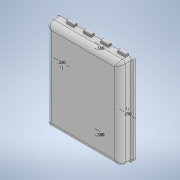
# Autodesk Inventor part: Top
Saved by Autodesk Inventor 2022 (Build 260153000, 153)
## iProperties
Created: 2022-03-05
Part Number: Top
Material: Generic
Document SubType Name: Modeling
Designer: Stump
Density: 1 g/cm^3
Appearance: Default
Author: Stump
Autodesk Inventor part; units mm, degrees
ref_plane "XZ Plane" through (0, 0, 0) normal (0, 1, 0) x (-1, 0, 0)
sketch "Sketch1" plane through (0, 0, 0) normal (0, 0, 1) x (1, 0, 0)
  line L0 (0, 0) -> (177.9524, 0)
  line L1 (177.9524, 0) -> (177.9524, 218.44)
  line L2 (177.9524, 218.44) -> (0, 218.44)
  line L3 (0, 218.44) -> (0, 0)
  line L4 (12.7, 205.74) -> (165.2524, 205.74)
  line L5 (165.2524, 205.74) -> (165.2524, 12.7)
  line L6 (165.2524, 12.7) -> (12.7, 12.7)
  line L7 (12.7, 12.7) -> (12.7, 205.74)
  dimension "d0" = 177.9524
  dimension "d1" = 218.44
  dimension "d2" = 12.7
  constraints: 16 end point, 4 parallel, 2 perpendicular, 1 horizontal, 3 other
  measures "d0" distance of L2.end L1.end
  measures "d1" distance of L1.end L0.end
  measures "d2" distance between parallel lines of L2 L4
extrude "Extrusion1" add sketch "Sketch1" along normal blind 28.194
sketch "Sketch2" plane through (0, 0, 28.194) normal (0, 0, 1) x (1, 0, 0)
  line L0 (177.9524, 0) -> (177.9524, 218.44) projected
  line L1 (177.9524, 218.44) -> (0, 218.44) projected
  line L2 (0, 218.44) -> (0, 0) projected
  line L3 (0, 0) -> (177.9524, 0) projected
  line L4 (12.7, 205.74) -> (165.2524, 205.74) projected
  line L5 (165.2524, 205.74) -> (165.2524, 12.7) projected
  line L6 (165.2524, 12.7) -> (12.7, 12.7) projected
  line L7 (12.7, 12.7) -> (12.7, 205.74) projected
  line L8 (0, 218.44) -> (0, 0) projected
  line L9 (0, 0) -> (177.9524, 0) projected
  line L10 (0, 218.44) -> (177.9524, 218.44)
  line L11 (177.9524, 218.44) -> (177.9524, 0)
  line L12 (177.9524, 0) -> (0, 0)
  line L13 (0, 0) -> (0, 218.44)
  constraints: 8 end point, 2 parallel, 1 horizontal, 1 perpendicular
extrude "Extrusion2" add sketch "Sketch2" against normal blind 3.175 contours L4 L5 L6 L7
fillet "Fillet1" radius 3.175 4 edges at (88.9762, 205.74, 25.019) (165.2524, 109.22, 25.019) (88.9762, 12.7, 25.019) (12.7, 109.22, 25.019)
fillet "Fillet3" radius 12.7 4 edges at (88.9762, 218.44, 28.194) (177.9524, 109.22, 28.194) (88.9762, 0, 28.194) (0, 109.22, 28.194)
fillet "Fillet4" radius 6.35 8 edges at (3.7197, 3.7197, 24.4743) (0, 0, 7.747) (174.2327, 3.7197, 24.4743) (177.9524, 0, 7.747) (3.7197, 214.7203, 24.4743) (0, 218.44, 7.747) (174.2327, 214.7203, 24.4743) (177.9524, 218.44, 7.747)
sketch "Sketch4" plane through (0, 0, 0) normal (0, 0, -1) x (-1, 0, 0)
  arc A0 (-177.9524, 6.35) -> (-171.6024, 0) centre (-171.6024, 6.35) ccw projected
  line L0 (0, 212.09) -> (0, 6.35) projected
  line L1 (0, 6.35) -> (0, 212.09)
  line L2 (-177.9524, 212.09) -> (-177.9524, 6.35)
  arc A1 (-171.6024, 218.44) -> (-177.9524, 212.09) centre (-171.6024, 212.09) ccw projected
  arc A2 (-171.6024, 218.44) -> (-177.9524, 212.09) centre (-171.6024, 212.09) ccw
  arc A3 (0, 212.09) -> (-6.35, 218.44) centre (-6.35, 212.09) ccw projected
  line L3 (-171.6024, 218.44) -> (-6.35, 218.44) projected
  arc A4 (0, 212.09) -> (-6.35, 218.44) centre (-6.35, 212.09) ccw
  line L4 (-177.9524, 6.35) -> (-177.9524, 212.09) projected
  line L5 (-6.35, 0) -> (-171.6024, 0) projected
  arc A5 (-177.9524, 6.35) -> (-171.6024, 0) centre (-171.6024, 6.35) ccw
  arc A6 (-6.35, 0) -> (0, 6.35) centre (-6.35, 6.35) ccw projected
  arc A7 (-6.35, 0) -> (0, 6.35) centre (-6.35, 6.35) ccw
  line L6 (-171.6024, 0) -> (-6.35, 0)
  line L7 (-6.35, 218.44) -> (-171.6024, 218.44)
  line L8 (-177.9524, 212.09) -> (-177.9524, 6.35)
  arc A8 (-171.6024, 221.615) -> (-181.1274, 212.09) centre (-171.6024, 212.09) ccw
  line L9 (-171.6024, 221.615) -> (-6.35, 221.615)
  arc A9 (3.175, 212.09) -> (-6.35, 221.615) centre (-6.35, 212.09) ccw
  line L10 (3.175, 212.09) -> (3.175, 6.35)
  arc A10 (-6.35, -3.175) -> (3.175, 6.35) centre (-6.35, 6.35) ccw
  line L11 (-6.35, -3.175) -> (-171.6024, -3.175)
  arc A11 (-181.1274, 6.35) -> (-171.6024, -3.175) centre (-171.6024, 6.35) ccw
  line L12 (-181.1274, 6.35) -> (-181.1274, 212.09)
  line L13 (-177.9524, 212.09) -> (-181.1274, 212.09)
  line L14 (0, 212.09) -> (0, 6.35) projected
  line L15 (0, 212.09) -> (3.175, 212.09)
  point P0 (0, 0)
  dimension "d14" = 3.175
  constraints: 22 end point, 16 point on circle, 8 centre point, 5 equal length, 2 tangent, 1 perpendicular, 7 other
  measures "d14" distance between parallel lines of L4 L12
sketch "Sketch5" plane through (0, 0, 0) normal (0, 0, -1) x (-1, 0, 0)
  line L0 (-12.7, 205.74) -> (-165.2524, 205.74) projected
  line L1 (-88.9762, 205.74) -> (-88.9762, 193.04)
  line L2 (-165.2524, 12.7) -> (-12.7, 12.7) projected
  line L3 (-88.9762, 12.7) -> (-88.9762, 25.4)
  line L4 (-165.2524, 205.74) -> (-165.2524, 12.7) projected
  line L5 (-165.2524, 109.22) -> (-171.6024, 109.22)
  line L6 (-12.7, 12.7) -> (-12.7, 205.74) projected
  line L7 (-12.7, 109.22) -> (-6.35, 109.22)
  line L8 (-171.6024, 193.04) -> (-6.35, 193.04)
  line L9 (-6.35, 193.04) -> (-6.35, 25.4)
  line L10 (-6.35, 25.4) -> (-171.6024, 25.4)
  line L11 (-171.6024, 25.4) -> (-171.6024, 193.04)
  point P0 (0, 0)
  dimension "d17" = 12.7
  dimension "d18" = 12.7
  dimension "d19" = 6.35
  dimension "d20" = 6.35
  constraints: 16 end point, 4 midpoint, 3 horizontal, 2 parallel, 2 vertical, 1 perpendicular
  measures "d17" distance of L1.start L1.end
  measures "d18" distance of L3.start L3.end
  measures "d19" distance of L5.start L5.end
  measures "d20" distance of L7.start L7.end
ref_plane "Work Plane1" through (6.35, 0, 0) normal (1, 0, 0) x (0, 1, 0)
ref_plane "Work Plane2" through (171.45, 0, 0) normal (1, 0, 0) x (0, 1, 0)
ref_plane "Work Plane5" through (130.175, 0, 0) normal (1, 0, 0) x (0, 1, 0)
ref_plane "Work Plane4" through (88.9, 0, 0) normal (1, 0, 0) x (0, 1, 0)
sketch "Sketch6" plane through (6.35, 0, 0) normal (1, 0, 0) x (0, 1, 0)
  line L0 (218.44, 0) -> (218.44, -6.35) projected
  line L1 (218.44, 0) -> (224.79, 0)
  line L2 (212.09, 0) -> (221.615, 0) projected
  line L3 (224.79, 0) -> (224.79, -6.35)
  line L4 (221.615, 0) -> (221.615, -6.35) projected
  line L5 (221.615, 0) -> (218.44, 0)
  line L6 (218.44, 0) -> (218.44, -6.35)
  line L7 (218.44, -6.35) -> (221.615, -6.35)
  line L8 (221.615, -6.35) -> (221.615, 0)
  point P0 (0, 0)
  dimension "d26" = 6.35
  dimension "d27" = 6.35
  constraints: 12 end point, 2 parallel, 2 perpendicular, 1 collinear, 1 horizontal
  measures "d26" distance of L0.start L1.end
  measures "d27" distance of L1.end L3.end
extrude "Extrusion5" cut sketch "Sketch6" along normal blind 165.1
sketch "Sketch14" plane through (171.45, 0, 0) normal (1, 0, 0) x (0, 1, 0)
  line L0 (218.44, 15.494) -> (218.44, 0) projected
  line L1 (218.44, 0) -> (224.79, 0)
  line L2 (224.79, 0) -> (224.79, 6.35)
  circle A0 centre (221.615, 3.175) radius 3.175
  circle A1 centre (221.615, 3.175) radius 1.5875
  point P0 (0, 0)
  dimension "d58" = 6.35
  dimension "d59" = 6.35
  dimension "d60" = 3.175
  constraints: 4 end point, 2 centre point, 1 coincident, 1 horizontal, 1 perpendicular
  measures "d58" distance of L0.end L1.end
  measures "d59" distance of L1.end L2.end
  measures "d60" diameter of A1
sketch "Sketch15" plane through (130.175, 0, 0) normal (1, 0, 0) x (0, 1, 0)
  line L0 (218.44, 15.494) -> (218.44, 0) projected
  line L1 (218.44, 0) -> (224.79, 0)
  line L2 (224.79, 0) -> (224.79, 6.35)
  line L3 (218.44, 0) -> (221.615, 0) projected
  circle A0 centre (221.615, 3.175) radius 3.175
  circle A1 centre (221.615, 3.175) radius 1.5875
  point P0 (0, 0)
  dimension "d61" = 6.35
  dimension "d62" = 6.35
  dimension "d63" = 3.175
  constraints: 4 end point, 1 centre point, 1 coincident, 1 horizontal, 1 perpendicular, 1 vertical alignment, 2 other
  measures "d61" distance of L0.end L1.end
  measures "d62" distance of L1.end L2.end
  measures "d63" diameter of A1
sketch "Sketch16" plane through (88.9, 0, 0) normal (1, 0, 0) x (0, 1, 0)
  line L0 (218.44, 15.494) -> (218.44, 0) projected
  line L1 (218.44, 0) -> (224.79, 0)
  line L2 (224.79, 0) -> (224.79, 6.35)
  circle A0 centre (221.615, 3.175) radius 3.175
  circle A1 centre (221.615, 3.175) radius 1.5875
  point P0 (0, 0)
  dimension "d64" = 6.35
  dimension "d65" = 6.35
  dimension "d66" = 3.175
  constraints: 4 end point, 2 centre point, 1 coincident, 1 horizontal, 1 perpendicular
  measures "d64" distance of L0.end L1.end
  measures "d65" distance of L1.end L2.end
  measures "d66" diameter of A1
sketch "Sketch17" plane through (47.625, 0, 0) normal (1, 0, 0) x (0, 1, 0)
  line L0 (218.44, 15.494) -> (218.44, 0) projected
  line L1 (218.44, 0) -> (224.79, 0)
  line L2 (224.79, 0) -> (224.79, 6.35)
  line L3 (218.44, 0) -> (221.615, 0) projected
  circle A0 centre (221.615, 3.175) radius 3.175
  circle A1 centre (221.615, 3.175) radius 1.5875
  point P0 (0, 0)
  dimension "d67" = 6.35
  dimension "d68" = 6.35
  dimension "d69" = 3.175
  constraints: 4 end point, 1 centre point, 1 coincident, 1 horizontal, 1 perpendicular, 1 vertical alignment, 2 other
  measures "d67" distance of L0.end L1.end
  measures "d68" distance of L1.end L2.end
  measures "d69" diameter of A1
extrude "Extrusion12" add sketch "Sketch14" against normal blind 19.3675 contours A0
extrude "Extrusion13" add sketch "Sketch15" against normal blind 19.3675 contours A0
extrude "Extrusion14" add sketch "Sketch16" against normal blind 19.3675 contours A0
extrude "Extrusion15" add sketch "Sketch17" against normal blind 19.3675 contours A0
sketch "Sketch18" plane through (171.45, 0, 0) normal (1, 0, 0) x (0, 1, 0)
  line L0 (221.615, 5.0743) -> (219.6994, 5.0743)
  line L1 (216.535, 5.0743) -> (216.535, 8.2493)
  line L2 (216.535, 8.2493) -> (221.615, 8.2493)
  line L3 (221.615, 8.2493) -> (221.615, 5.0743)
  line L4 (216.535, 8.2493) -> (219.6994, 8.2493)
  line L5 (219.6994, 5.0743) -> (219.6994, 3.175)
  line L6 (219.6994, 3.175) -> (216.535, 3.175)
  line L7 (216.535, 3.175) -> (216.535, 8.2493)
  point P0 (0, 0)
  dimension "d78" = 5.08
  dimension "d79" = 3.175
  constraints: 16 end point, 4 parallel, 2 horizontal, 2 perpendicular
  measures "d78" distance of L1.end L2.end
  measures "d79" distance of L1.start L1.end
extrude "Extrusion16" add sketch "Sketch18" against normal blind 141.9225
sketch "Sketch19" plane through (152.0825, 219.6994, 3.175) normal (0, 0, -1) x (-1, 0, 0)
  line L0 (21.9075, 0) -> (21.9075, -1.2594) projected
  line L1 (0, 0) -> (21.9075, 0) projected
  line L2 (0, -1.2594) -> (0, 0) projected
  line L3 (21.9075, -1.2594) -> (0, -1.2594) projected
  line L4 (0, 1.9156) -> (21.9075, 1.9156) projected
  line L5 (63.1825, 0) -> (63.1825, -1.2594) projected
  line L6 (41.275, 0) -> (63.1825, 0) projected
  line L7 (41.275, -1.2594) -> (41.275, 0) projected
  line L8 (63.1825, -1.2594) -> (41.275, -1.2594) projected
  line L9 (41.275, 1.9156) -> (63.1825, 1.9156) projected
  line L10 (104.4575, 0) -> (104.4575, -1.2594) projected
  line L11 (82.55, 0) -> (104.4575, 0) projected
  line L12 (82.55, -1.2594) -> (82.55, 0) projected
  line L13 (104.4575, -1.2594) -> (82.55, -1.2594) projected
  line L14 (82.55, 1.9156) -> (104.4575, 1.9156) projected
  line L15 (0, -1.2594) -> (21.9075, -1.2594)
  line L16 (21.9075, -1.2594) -> (21.9075, 1.9156)
  line L17 (21.9075, 1.9156) -> (0, 1.9156)
  line L18 (0, 1.9156) -> (0, -1.2594)
  line L19 (21.9075, -1.2594) -> (41.275, -1.2594) projected
  line L20 (41.275, -1.2594) -> (63.1825, -1.2594)
  line L21 (63.1825, -1.2594) -> (63.1825, 1.9156)
  line L22 (63.1825, 1.9156) -> (41.275, 1.9156)
  line L23 (41.275, 1.9156) -> (41.275, -1.2594)
  line L24 (104.4575, -1.2594) -> (82.55, -1.2594) projected
  line L25 (82.55, -1.2594) -> (104.4575, -1.2594)
  line L26 (104.4575, -1.2594) -> (104.4575, 1.9156)
  line L27 (104.4575, 1.9156) -> (82.55, 1.9156)
  line L28 (82.55, 1.9156) -> (82.55, -1.2594)
  point P0 (152.0825, -219.6994)
  constraints: 24 end point, 6 parallel, 3 horizontal, 3 perpendicular
extrude "Extrusion17" cut sketch "Sketch19" against normal blind 6.35
extrude "Extrusion18" add sketch "Sketch4" along normal blind 6.35 contours A0 L5 A6 L0 L15 L10 A10 L11 A11 L12 L13 L2
sketch "Sketch22" plane through (0, 0, 0) normal (0, 0, 1) x (1, 0, 0)
  arc A0 (0, 6.35) -> (6.35, 0) centre (6.35, 6.35) ccw projected
  arc A1 (-3.175, 6.35) -> (6.35, -3.175) centre (6.35, 6.35) ccw projected
  line L0 (171.6024, -3.175) -> (6.35, -3.175) projected
  line L1 (171.6024, 0) -> (165.2524, 12.7) projected
  line L2 (177.9524, 6.35) -> (177.9524, 212.09) projected
  line L3 (181.1274, 212.09) -> (181.1274, 6.35) projected
  arc A2 (171.6024, -3.175) -> (181.1274, 6.35) centre (171.6024, 6.35) ccw projected
  arc A3 (171.6024, -3.175) -> (181.1274, 6.35) centre (171.6024, 6.35) ccw
  line L4 (-3.175, 6.35) -> (-3.175, 212.09) projected
  arc A4 (-3.175, 6.35) -> (6.35, -3.175) centre (6.35, 6.35) ccw
  line L5 (6.35, 0) -> (171.6024, 0) projected
  line L6 (6.35, -3.175) -> (171.6024, -3.175)
  line L7 (171.6024, 0) -> (6.35, 0)
  line L8 (177.9524, 6.35) -> (177.9524, 212.09)
  line L9 (177.9524, 212.09) -> (181.1274, 212.09)
  line L10 (181.1274, 212.09) -> (181.1274, 6.35)
  line L11 (0, 212.09) -> (0, 6.35) projected
  line L12 (0, 6.35) -> (0, 212.09)
  line L13 (0, 212.09) -> (-3.175, 212.09)
  line L14 (-3.175, 212.09) -> (-3.175, 6.35)
  arc A5 (171.6024, 0) -> (177.9524, 6.35) centre (171.6024, 6.35) ccw projected
  arc A6 (171.6024, 0) -> (177.9524, 6.35) centre (171.6024, 6.35) ccw
  line L15 (171.6024, 0) -> (6.35, 0)
  arc A7 (0, 6.35) -> (6.35, 0) centre (6.35, 6.35) ccw
  point P0 (0, 0)
  constraints: 18 end point, 9 point on circle, 6 tangent, 4 centre point, 4 equal length, 1 concentric, 1 horizontal
extrude "Extrusion21" add sketch "Sketch22" along normal blind 2.54
chamfer "Chamfer2" distance 3.175 angle 45 5 edges at (88.9762, -3.175, 2.54) (178.3376, -0.3852, 2.54) (181.1274, 109.22, 2.54) (-0.3852, -0.3852, 2.54) (-3.175, 109.22, 2.54)
ref_plane "Work Plane3" through (47.625, 0, 0) normal (1, 0, 0) x (0, 1, 0)
body "Solid1"
